Autodesk Inventor part; units mm, degrees
(part 2 of 2)
  spline S446 degree 2 poles (2.6508, -5.4084) (2.6868, -5.3964) (2.7198, -5.3964) knots 0 0 0 1 1 1
  spline S447 degree 2 poles (2.7198, -5.3964) (2.8579, -5.3964) (2.9059, -5.5405) knots 0 0 0 1 1 1
  spline S448 degree 2 poles (2.9059, -5.5405) (2.9119, -5.5585) (2.9149, -5.5915) knots 0 0 0 1 1 1
  spline S449 degree 2 poles (2.9149, -5.5915) (2.9149, -5.6996) (2.8039, -5.7656) knots 0 0 0 1 1 1
  spline S450 degree 2 poles (2.8039, -5.7656) (2.7288, -5.7837) (2.4557, -5.8077) knots 0 0 0 1 1 1
  spline S451 degree 2 poles (2.4557, -5.8077) (2.5127, -6.1949) (2.5127, -6.8763) knots 0 0 0 1 1 1
  spline S452 degree 2 poles (2.5127, -6.8763) (2.5127, -7.1554) (2.4917, -8.3201) knots 0 0 0 1 1 1
  line L95 (2.4917, -8.3201) -> (2.4917, -8.3651)
  spline S453 degree 2 poles (2.4917, -8.3651) (2.7678, -8.3531) (2.8009, -8.3441) knots 0 0 0 1 1 1
  spline S454 degree 2 poles (2.8009, -8.3441) (2.9239, -8.3441) (2.984, -8.4762) knots 0 0 0 1 1 1
  spline S455 degree 2 poles (2.984, -8.4762) (2.996, -8.5122) (2.996, -8.5392) knots 0 0 0 1 1 1
  line L96 (2.996, -8.5392) -> (2.996, -8.5422)
  spline S456 degree 2 poles (2.996, -8.5422) (2.996, -8.6743) (2.8519, -8.7313) knots 0 0 0 1 1 1
  spline S457 degree 2 poles (2.8519, -8.7313) (2.7378, -8.7433) (1.8193, -8.7824) knots 0 0 0 1 1 1
  spline S458 degree 2 poles (1.8193, -8.7824) (1.7112, -8.7824) (1.6482, -8.6713) knots 0 0 0 1 1 1
  spline S459 degree 2 poles (1.6482, -8.6713) (1.6302, -8.6323) (1.6302, -8.5903) knots 0 0 0 1 1 1
  line L97 (1.6302, -8.5903) -> (1.6302, -8.5812)
  spline S460 degree 2 poles (1.6302, -8.5812) (1.6302, -8.4762) (1.7413, -8.4132) knots 0 0 0 1 1 1
  spline S461 degree 2 poles (1.7413, -8.4132) (1.7743, -8.3891) (1.9664, -8.3891) knots 0 0 0 1 1 1
  spline S462 degree 2 poles (1.9664, -8.3891) (1.9664, -8.3861) (2.0985, -8.3831) knots 0 0 0 1 1 1
  spline S463 degree 2 poles (2.0985, -8.3831) (2.1255, -7.2455) (2.1255, -6.9663) knots 0 0 0 1 1 1
  line L98 (2.1255, -6.9663) -> (2.1255, -6.7832)
  spline S464 degree 2 poles (2.1255, -6.7832) (2.1255, -6.1889) (2.0654, -5.8347) knots 0 0 0 1 1 1
  spline S465 degree 2 poles (2.0654, -5.8347) (2.0474, -5.8347) (1.6572, -5.8647) knots 0 0 0 1 1 1
  spline S466 degree 2 poles (1.6572, -5.8647) (1.5672, -5.8647) (1.4981, -5.7776) knots 0 0 0 1 1 1
  spline S467 degree 2 poles (1.4981, -5.7776) (1.4681, -5.7266) (1.4681, -5.6786) knots 0 0 0 1 1 1
  line L99 (1.4681, -5.6786) -> (1.4681, -5.6606)
  spline S468 degree 2 poles (1.4681, -5.6606) (1.4681, -5.5615) (1.5732, -5.4985) knots 0 0 0 1 1 1
  spline S469 degree 2 poles (1.5732, -5.4985) (1.6182, -5.4745) (1.6842, -5.4715) knots 0 0 0 1 1 1
  spline S470 degree 2 poles (1.6842, -5.4715) (1.9754, -5.4535) (1.9964, -5.4505) knots 0 0 0 1 1 1
  spline S471 degree 2 poles (1.9964, -5.4505) (1.9964, -5.3994) (2.0654, -5.3304) knots 0 0 0 1 1 1
  spline S472 degree 2 poles (2.0654, -5.3304) (2.1285, -5.2914) (2.1705, -5.2914) knots 0 0 0 1 1 1
  line L100 (5.2623, -5.3994) -> (5.2953, -5.3994)
  spline S473 degree 2 poles (5.2953, -5.3994) (5.3733, -5.3994) (5.4454, -5.4925) knots 0 0 0 1 1 1
  spline S474 degree 2 poles (5.4454, -5.4925) (5.4784, -5.5345) (5.4784, -5.7236) knots 0 0 0 1 1 1
  spline S475 degree 2 poles (5.4784, -5.7236) (5.5024, -6.381) (5.5024, -6.9333) knots 0 0 0 1 1 1
  line L101 (5.5024, -6.9333) -> (5.5024, -6.9603)
  spline S476 degree 2 poles (5.5024, -6.9603) (5.5024, -8.215) (5.3343, -8.5302) knots 0 0 0 1 1 1
  spline S477 degree 2 poles (5.3343, -8.5302) (5.2683, -8.6473) (5.1722, -8.6473) knots 0 0 0 1 1 1
  spline S478 degree 2 poles (5.1722, -8.6473) (4.9651, -8.6473) (4.746, -8.164) knots 0 0 0 1 1 1
  spline S479 degree 2 poles (4.746, -8.164) (4.6319, -7.9149) (4.3497, -7.2245) knots 0 0 0 1 1 1
  spline S480 degree 2 poles (4.3497, -7.2245) (4.1036, -6.6541) (3.8725, -6.2939) knots 0 0 0 1 1 1
  line L102 (3.8725, -6.2939) -> (3.8695, -6.2939)
  spline S481 degree 2 poles (3.8695, -6.2939) (3.8695, -6.342) (3.8665, -6.5161) knots 0 0 0 1 1 1
  line L103 (3.8665, -6.5161) -> (3.8755, -7.7047)
  spline S482 degree 2 poles (3.8755, -7.7047) (3.8755, -8.7614) (3.7284, -8.8484) knots 0 0 0 1 1 1
  spline S483 degree 2 poles (3.7284, -8.8484) (3.6744, -8.8964) (3.6143, -8.8964) knots 0 0 0 1 1 1
  line L104 (3.6143, -8.8964) -> (3.6053, -8.8964)
  spline S484 degree 2 poles (3.6053, -8.8964) (3.4732, -8.8964) (3.4192, -8.7553) knots 0 0 0 1 1 1
  spline S485 degree 2 poles (3.4192, -8.7553) (3.4102, -8.7223) (3.4102, -8.7013) knots 0 0 0 1 1 1
  spline S486 degree 2 poles (3.4102, -8.7013) (3.4102, -8.6803) (3.4432, -8.5452) knots 0 0 0 1 1 1
  spline S487 degree 2 poles (3.4432, -8.5452) (3.4883, -8.3021) (3.4883, -7.7738) knots 0 0 0 1 1 1
  line L105 (3.4883, -7.7738) -> (3.4883, -7.6927)
  spline S488 degree 2 poles (3.4883, -7.6927) (3.4883, -7.4706) (3.4793, -6.7592) knots 0 0 0 1 1 1
  spline S489 degree 2 poles (3.4793, -6.7592) (3.4793, -5.9157) (3.6173, -5.7867) knots 0 0 0 1 1 1
  spline S490 degree 2 poles (3.6173, -5.7867) (3.7074, -5.7026) (3.7854, -5.7026) knots 0 0 0 1 1 1
  spline S491 degree 2 poles (3.7854, -5.7026) (3.9265, -5.7026) (4.1096, -5.9577) knots 0 0 0 1 1 1
  spline S492 degree 2 poles (4.1096, -5.9577) (4.2897, -6.2039) (4.4668, -6.5551) knots 0 0 0 1 1 1
  spline S493 degree 2 poles (4.4668, -6.5551) (4.704, -7.0414) (5.0491, -7.8969) knots 0 0 0 1 1 1
  spline S494 degree 2 poles (5.0491, -7.8969) (5.1002, -8.0169) (5.1242, -8.0379) knots 0 0 0 1 1 1
  line L106 (5.1242, -8.0379) -> (5.1332, -8.0379)
  spline S495 degree 2 poles (5.1332, -8.0379) (5.1422, -7.9209) (5.1422, -7.7528) knots 0 0 0 1 1 1
  spline S496 degree 2 poles (5.1422, -7.7528) (5.1422, -7.1464) (5.0852, -5.5885) knots 0 0 0 1 1 1
  spline S497 degree 2 poles (5.0852, -5.5885) (5.0852, -5.4895) (5.1932, -5.4204) knots 0 0 0 1 1 1
  spline S498 degree 2 poles (5.1932, -5.4204) (5.2383, -5.3994) (5.2623, -5.3994) knots 0 0 0 1 1 1
  line L107 (7.2314, -5.3004) -> (7.2434, -5.3004)
  spline S499 degree 2 poles (7.2434, -5.3004) (7.5946, -5.3004) (7.8828, -5.5525) knots 0 0 0 1 1 1
  spline S500 degree 2 poles (7.8828, -5.5525) (8.0208, -5.6876) (8.0749, -5.7837) knots 0 0 0 1 1 1
  spline S501 degree 2 poles (8.0749, -5.7837) (8.228, -6.0538) (8.228, -6.351) knots 0 0 0 1 1 1
  spline S502 degree 2 poles (8.228, -6.351) (8.228, -6.459) (8.1229, -6.5221) knots 0 0 0 1 1 1
  spline S503 degree 2 poles (8.1229, -6.5221) (8.0779, -6.5431) (8.0329, -6.5431) knots 0 0 0 1 1 1
  spline S504 degree 2 poles (8.0329, -6.5431) (7.9068, -6.5431) (7.8528, -6.414) knots 0 0 0 1 1 1
  spline S505 degree 2 poles (7.8528, -6.414) (7.8437, -6.414) (7.8317, -6.2369) knots 0 0 0 1 1 1
  spline S506 degree 2 poles (7.8317, -6.2369) (7.8047, -6.1048) (7.7687, -6.0358) knots 0 0 0 1 1 1
  spline S507 degree 2 poles (7.7687, -6.0358) (7.7357, -5.9577) (7.6276, -5.8467) knots 0 0 0 1 1 1
  spline S508 degree 2 poles (7.6276, -5.8467) (7.4445, -5.6906) (7.2494, -5.6906) knots 0 0 0 1 1 1
  line L108 (7.2494, -5.6906) -> (7.2284, -5.6906)
  spline S509 degree 2 poles (7.2284, -5.6906) (6.9432, -5.6906) (6.6941, -6.0058) knots 0 0 0 1 1 1
  spline S510 degree 2 poles (6.6941, -6.0058) (6.595, -6.1529) (6.544, -6.2729) knots 0 0 0 1 1 1
  spline S511 degree 2 poles (6.544, -6.2729) (6.463, -6.456) (6.3939, -6.7892) knots 0 0 0 1 1 1
  spline S512 degree 2 poles (6.3939, -6.7892) (6.3399, -7.1284) (6.3399, -7.4016) knots 0 0 0 1 1 1
  line L109 (6.3399, -7.4016) -> (6.3399, -7.4346)
  spline S513 degree 2 poles (6.3399, -7.4346) (6.3399, -8.077) (6.6431, -8.3441) knots 0 0 0 1 1 1
  spline S514 degree 2 poles (6.6431, -8.3441) (6.8142, -8.4882) (7.0603, -8.4882) knots 0 0 0 1 1 1
  spline S515 degree 2 poles (7.0603, -8.4882) (7.4445, -8.4882) (7.8407, -8.191) knots 0 0 0 1 1 1
  spline S516 degree 2 poles (7.8407, -8.191) (8.0539, -8.0169) (8.1079, -7.8188) knots 0 0 0 1 1 1
  spline S517 degree 2 poles (8.1079, -7.8188) (8.1139, -7.7798) (8.1139, -7.7678) knots 0 0 0 1 1 1
  spline S518 degree 2 poles (8.1139, -7.7678) (8.1139, -7.5337) (7.6606, -7.4016) knots 0 0 0 1 1 1
  spline S519 degree 2 poles (7.6606, -7.4016) (7.5166, -7.4526) (7.5166, -7.5126) knots 0 0 0 1 1 1
  spline S520 degree 2 poles (7.5166, -7.5126) (7.4775, -7.5907) (7.3965, -7.6207) knots 0 0 0 1 1 1
  spline S521 degree 2 poles (7.3965, -7.6207) (7.3605, -7.6297) (7.3485, -7.6297) knots 0 0 0 1 1 1
  line L110 (7.3485, -7.6297) -> (7.3214, -7.6297)
  spline S522 degree 2 poles (7.3214, -7.6297) (7.2254, -7.6297) (7.1624, -7.5216) knots 0 0 0 1 1 1
  spline S523 degree 2 poles (7.1624, -7.5216) (7.1413, -7.4736) (7.1413, -7.4316) knots 0 0 0 1 1 1
  spline S524 degree 2 poles (7.1413, -7.4316) (7.1413, -7.3235) (7.2794, -7.1794) knots 0 0 0 1 1 1
  spline S525 degree 2 poles (7.2794, -7.1794) (7.4295, -7.0504) (7.6756, -6.9873) knots 0 0 0 1 1 1
  spline S526 degree 2 poles (7.6756, -6.9873) (7.9278, -6.9333) (8.1829, -6.9333) knots 0 0 0 1 1 1
  line L111 (8.1829, -6.9333) -> (8.231, -6.9333)
  spline S527 degree 2 poles (8.231, -6.9333) (8.4081, -6.9333) (8.4411, -6.9573) knots 0 0 0 1 1 1
  spline S528 degree 2 poles (8.4411, -6.9573) (8.5431, -7.0264) (8.5431, -7.1344) knots 0 0 0 1 1 1
  spline S529 degree 2 poles (8.5431, -7.1344) (8.5431, -7.2515) (8.4201, -7.3145) knots 0 0 0 1 1 1
  spline S530 degree 2 poles (8.4201, -7.3145) (8.4051, -7.3205) (8.351, -7.3265) knots 0 0 0 1 1 1
  line L112 (8.351, -7.3265) -> (8.336, -7.3235)
  line L113 (8.336, -7.3235) -> (8.33, -7.3235)
  spline S531 degree 2 poles (8.33, -7.3235) (8.5041, -7.5126) (8.5041, -7.7288) knots 0 0 0 1 1 1
  line L114 (8.5041, -7.7288) -> (8.5041, -7.7648)
  spline S532 degree 2 poles (8.5041, -7.7648) (8.5041, -8.0049) (8.303, -8.2661) knots 0 0 0 1 1 1
  spline S533 degree 2 poles (8.303, -8.2661) (8.1439, -8.4552) (8.0389, -8.5272) knots 0 0 0 1 1 1
  spline S534 degree 2 poles (8.0389, -8.5272) (7.8678, -8.6533) (7.7087, -8.7253) knots 0 0 0 1 1 1
  spline S535 degree 2 poles (7.7087, -8.7253) (7.3665, -8.8754) (7.0933, -8.8754) knots 0 0 0 1 1 1
  line L115 (7.0933, -8.8754) -> (7.0213, -8.8754)
  spline S536 degree 2 poles (7.0213, -8.8754) (6.7541, -8.8754) (6.496, -8.7283) knots 0 0 0 1 1 1
  spline S537 degree 2 poles (6.496, -8.7283) (6.2108, -8.5602) (6.0667, -8.176) knots 0 0 0 1 1 1
  spline S538 degree 2 poles (6.0667, -8.176) (5.9497, -7.8578) (5.9497, -7.4616) knots 0 0 0 1 1 1
  line L116 (5.9497, -7.4616) -> (5.9497, -7.3806)
  spline S539 degree 2 poles (5.9497, -7.3806) (5.9497, -6.9453) (6.0697, -6.456) knots 0 0 0 1 1 1
  spline S540 degree 2 poles (6.0697, -6.456) (6.1598, -6.1619) (6.2588, -5.9788) knots 0 0 0 1 1 1
  spline S541 degree 2 poles (6.2588, -5.9788) (6.3339, -5.8257) (6.481, -5.6606) knots 0 0 0 1 1 1
  spline S542 degree 2 poles (6.481, -5.6606) (6.616, -5.5165) (6.6971, -5.4685) knots 0 0 0 1 1 1
  spline S543 degree 2 poles (6.6971, -5.4685) (6.9552, -5.3004) (7.2314, -5.3004) knots 0 0 0 1 1 1
  point P0 (0, 0)
  constraints: 2 other
sketch "Sketch2" plane through (0, 0, 0) normal (0, 0, 1) x (1, 0, 0)
  arc A0 (9.1546, 1.5914) -> (8.9503, 1.4908) centre (9.0672, 1.5111) ccw
  arc A1 (6.2006, -3.4936) -> (6.3784, -3.3211) centre (6.2717, -3.3891) ccw
  arc A2 (8.3263, -3.2626) -> (8.3973, -3.534) centre (8.3973, -3.389) ccw
  arc A3 (8.3403, 1.9046) -> (6.7092, 3.7431) centre (6.452, 1.8721) ccw
  arc A4 (8.3403, 1.0769) -> (8.8699, 0.9191) centre (8.6289, 1.0777) ccw
  arc A5 (8.3973, -3.534) -> (10.0494, -1.9367) centre (7.9149, -1.382) ccw
  arc A6 (8.3263, -3.2626) -> (8.3403, -1.697) centre (7.7459, -2.4745) ccw
  arc A7 (7.4463, -0.2993) -> (8.3403, -1.697) centre (9.2937, -0.1024) ccw
  arc A8 (4.9393, 0.3254) -> (6.2717, -3.5155) centre (6.9699, -1.1217) ccw
  arc A9 (4.9393, 0.3254) -> (6.3432, 2.0448) centre (-5.6011, 10.3652) ccw
  arc A10 (6.3432, 2.0448) -> (6.612, 3.6157) centre (5.1128, 3.0638) ccw
  arc A11 (8.3403, 1.9046) -> (8.3403, 1.0769) centre (14.4531, 1.4906) ccw
  arc A12 (8.9175, 0.9991) -> (8.9503, 1.4908) centre (7.9785, 1.3088) ccw
  arc A13 (10.0494, -1.9367) -> (9.1546, 1.5914) centre (5.3594, -1.2487) ccw
  arc A14 (8.8699, 0.9191) -> (8.9175, 0.9991) centre (8.7464, 1.0466) ccw
  arc A15 (6.7092, 3.7431) -> (6.612, 3.6157) centre (6.6878, 3.6587) ccw
  arc A16 (6.685, -1.2554) -> (6.3164, -1.6748) centre (7.275, -2.1455) ccw
  arc A17 (6.685, -1.2554) -> (7.4485, -0.3185) centre (5.5611, 0.4399) ccw
  arc A18 (6.2717, -3.1424) -> (6.3784, -3.3211) centre (6.7043, -3.0055) ccw
  arc A19 (6.3164, -1.6748) -> (6.2717, -3.1424) centre (7.9111, -2.4578) ccw
  arc A20 (-4.0564, 1.588) -> (-4.2607, 1.4873) centre (-4.1438, 1.5077) ccw
  arc A21 (-7.0104, -3.497) -> (-6.8326, -3.3245) centre (-6.9393, -3.3925) ccw
  arc A22 (-4.8847, -3.266) -> (-4.8137, -3.5375) centre (-4.8137, -3.3925) ccw
  arc A23 (-4.8707, 1.9011) -> (-6.5018, 3.7397) centre (-6.759, 1.8687) ccw
  arc A24 (-4.8707, 1.0735) -> (-4.3411, 0.9156) centre (-4.5821, 1.0743) ccw
  arc A25 (-4.8137, -3.5375) -> (-3.1616, -1.9401) centre (-5.2961, -1.3854) ccw
  arc A26 (-4.8847, -3.266) -> (-4.8707, -1.7004) centre (-5.4651, -2.478) ccw
  arc A27 (-5.7647, -0.3027) -> (-4.8707, -1.7004) centre (-3.9173, -0.1059) ccw
  arc A28 (-8.2717, 0.322) -> (-6.9393, -3.5189) centre (-6.2411, -1.1251) ccw
  arc A29 (-8.2717, 0.322) -> (-6.8678, 2.0413) centre (-18.8121, 10.3618) ccw
  arc A30 (-6.8678, 2.0413) -> (-6.599, 3.6123) centre (-8.0982, 3.0603) ccw
  arc A31 (-4.8707, 1.9011) -> (-4.8707, 1.0735) centre (1.2421, 1.4871) ccw
  arc A32 (-4.2935, 0.9956) -> (-4.2607, 1.4873) centre (-5.2325, 1.3053) ccw
  arc A33 (-3.1616, -1.9401) -> (-4.0564, 1.588) centre (-7.8516, -1.2521) ccw
  arc A34 (-4.3411, 0.9156) -> (-4.2935, 0.9956) centre (-4.4646, 1.0431) ccw
  arc A35 (-6.5018, 3.7397) -> (-6.599, 3.6123) centre (-6.5232, 3.6552) ccw
  arc A36 (-6.526, -1.2588) -> (-6.8946, -1.6782) centre (-5.936, -2.1489) ccw
  arc A37 (-6.526, -1.2588) -> (-5.7625, -0.3219) centre (-7.6499, 0.4365) ccw
  arc A38 (-6.9393, -3.1458) -> (-6.8326, -3.3245) centre (-6.5067, -3.0089) ccw
  arc A39 (-6.8946, -1.6782) -> (-6.9393, -3.1458) centre (-5.2999, -2.4613) ccw
  point P0 (0, 0)
  constraints: 98 point on circle, 40 centre point, 2 tangent
extrude "Extrusion1" add sketch "Sketch1" against normal blind 5
extrude "Extrusion2" add sketch "Sketch2" against normal blind 5 contours A13 A5 A2 A6 A7 A17 A16 A19 A18 A1 A8 A9 A10 A15 A3 A11 A4 A14 A12 A0 | A33 A25 A22 A26 A27 A37 A36 A39 A38 A21 A28 A29 A30 A35 A23 A31 A24 A34 A32 A20
sketch "Sketch4" plane through (0, 0, -5) normal (0, 0, -1) x (-1, 0, 0)
  line L0 (10.394, -11.982) -> (-10.8404, -11.982)
  line L1 (-12.8404, -9.982) -> (-12.8404, 9.1581)
  line L2 (-10.8404, 11.1581) -> (10.394, 11.1581)
  line L3 (12.394, 9.1581) -> (12.394, -9.982)
  arc A0 (12.394, 9.1581) -> (10.394, 11.1581) centre (10.394, 9.1581) ccw
  arc A1 (10.394, -11.982) -> (12.394, -9.982) centre (10.394, -9.982) ccw
  arc A2 (-12.8404, -9.982) -> (-10.8404, -11.982) centre (-10.8404, -9.982) ccw
  arc A3 (-10.8404, 11.1581) -> (-12.8404, 9.1581) centre (-10.8404, 9.1581) ccw
  point P0 (0, 0)
  dimension "d77" = 2
  constraints: 8 end point, 8 point on circle, 8 tangent, 4 centre point, 3 equal radius, 2 parallel, 1 horizontal, 1 perpendicular
  measures "d77" radius of A0
extrude "Extrusion3" add sketch "Sketch4" along normal blind 5
body "Solid1"
